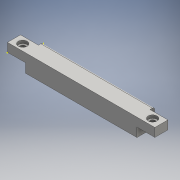
# Autodesk Inventor part: beam44mmVer2
Saved by Autodesk Inventor 2016 (Build 200138000, 138)
## iProperties
Created: 2015-11-25
Part Number: beam44mmVer2
Material: Generic
Document SubType Name: Modeling
Designer: hesaon
Density: 1 g/cm^3
Appearance: Default
Author: hesaon
Autodesk Inventor part; units mm, degrees
ref_plane "YZ Plane" through (0, 0, 0) normal (1, 0, 0) x (0, 1, 0)
ref_plane "XZ Plane" through (0, 0, 0) normal (0, 1, 0) x (-1, 0, 0)
ref_plane "XY Plane" through (0, 0, 0) normal (0, 0, 1) x (1, 0, 0)
sketch "Sketch1" plane through (0, 0, 0) normal (0, 0, 1) x (1, 0, 0)
  line L0 (0, 0) -> (100, 0)
  line L1 (100, 0) -> (100, 8.85)
  line L2 (87.85, 12) -> (12.15, 12)
  line L3 (0, 8.85) -> (0, 0)
  line L4 (12.15, 12) -> (12.15, 8.85)
  line L5 (12.15, 8.85) -> (0, 8.85)
  line L6 (87.85, 12) -> (87.85, 8.85)
  line L7 (87.85, 8.85) -> (100, 8.85)
  dimension "d6" = 100
  dimension "d7" = 3.15
  dimension "d8" = 3.15
  dimension "d9" = 12.15
  dimension "d10" = 12.15
  dimension "d11" = 8.85
  dimension "d12" = 8.85
  dimension "d13" = 12
  constraints: 16 end point, 2 parallel, 1 horizontal, 1 perpendicular
  measures "d6" distance of L0.end L0.start
  measures "d7" distance of L2.end L4.end
  measures "d8" distance of L6.end L2.start
  measures "d9" distance between parallel lines of L4 L3
  measures "d10" distance between parallel lines of L1 L6
  measures "d11" distance of L3.start L0.start
  measures "d12" distance of L1.end L0.end
  measures "d13" distance from line of L0 L2.end
extrude "Extrusion1" add sketch "Sketch1" along normal blind 6
sketch "Sketch2" plane through (0, 0, 0) normal (0, 0, -1) x (-1, 0, 0)
  line L0 (-87.85, 12) -> (-12.15, 12) projected
  line L1 (0, 0) -> (-100, 0) projected
  line L2 (-87.85, 12) -> (-12, 12)
  line L3 (-12, 12) -> (-12, 0)
  line L4 (-12, 0) -> (-87.85, 0)
  line L5 (-87.85, 0) -> (-87.85, 12)
  constraints: 8 end point, 2 parallel, 1 horizontal, 1 perpendicular, 1 point on line
extrude "Extrusion2" add sketch "Sketch2" along normal blind 6
sketch "Sketch3" plane through (0, 0, 0) normal (0, 0, -1) x (-1, 0, 0)
  circle A0 centre (-6, 4.35) radius 1.725
  line L0 (-12, 8.85) -> (0, 8.85) projected
  line L1 (0, 8.85) -> (0, 0) projected
  circle A1 centre (-94, 4.5) radius 1.725
  line L2 (-87.85, 0) -> (-100, 0) projected
  line L3 (-100, 0) -> (-100, 8.85) projected
  point P0 (-12, 9)
  dimension "d18" = 3.45
  dimension "d19" = 4.5
  dimension "d20" = 6
  dimension "d21" = 3.45
  dimension "d22" = 4.5
  dimension "d23" = 6
  constraints: 2 centre point, 1 other
  measures "d18" diameter of A0
  measures "d20" distance from line of L1 A0.centre
  measures "d21" diameter of A1
  measures "d22" distance from line of L2 A1.centre
  measures "d23" distance from line of L3 A1.centre
extrude "Extrusion3" cut sketch "Sketch3" against normal blind 4
sketch "Sketch4" plane through (0, 0, 6) normal (0, 0, 1) x (1, 0, 0)
  circle A0 centre (6, 4.35) radius 3
  line L0 (12.15, 8.85) -> (0, 8.85) projected
  line L1 (0, 8.85) -> (0, 0) projected
  circle A1 centre (94, 4.5) radius 1.725 projected
  circle A2 centre (94, 4.5) radius 3
  dimension "d26" = 6
  dimension "d27" = 4.5
  dimension "d28" = 6
  dimension "d29" = 6
  constraints: 2 centre point, 1 coincident
  measures "d26" diameter of A0
  measures "d27" distance from line of L0 A0.centre
  measures "d28" distance from line of L1 A0.centre
  measures "d29" diameter of A2
extrude "Extrusion4" cut sketch "Sketch4" against normal blind 2 contours A0 | A1 | A2
sketch "Sketch5" plane through (87.85, 0, 0) normal (0, -1, 0) x (1, 0, 0)
  point P0 (-87.85, 0)
sketch "Sketch6" plane through (0, 0, 0) normal (0, 0, -1) x (-1, 0, 0)
  line L0 (0, 0) -> (-100, 0) projected
  line L1 (-12.15, 8.85) -> (0, 8.85) projected
  line L2 (0, 0) -> (0, 8.85)
  line L3 (-12.15, 8.85) -> (-12, 8.85) projected
  line L4 (0, 8.85) -> (-12, 8.85)
  line L5 (-12, 0) -> (-12, 12) projected
  line L6 (-12, 8.85) -> (-12, 0)
  line L7 (-12, 0) -> (0, 0)
  line L8 (-100, 0) -> (-100, 8.85) projected
  line L9 (-100, 0) -> (-87.85, 0)
  line L10 (-87.85, 0) -> (-87.85, 8.85) projected
  line L11 (-87.85, 0) -> (-87.85, 8.85)
  line L12 (-87.85, 8.85) -> (-100, 8.85)
  line L13 (-100, 8.85) -> (-100, 0)
  dimension "d33" = 12.15
  constraints: 16 end point, 5 collinear, 1 perpendicular, 1 point on line, 1 vertical
  measures "d33" distance of L0.end L9.end
extrude "Extrusion5" cut sketch "Sketch6" against normal blind 0.15
sketch "Sketch7" plane through (12, 8.85, 0) normal (-1, 0, 0) x (0, 0, 1)
  line L0 (0, 3.15) -> (0, 0) projected
  line L1 (0, 3.15) -> (0, 0)
  line L2 (0.15, 0) -> (6, 0) projected
  line L3 (0, 0) -> (0.15, 0)
  line L4 (0.15, 0) -> (0.15, -8.85) projected
  line L5 (0.15, 0) -> (0.15, -8.85)
  line L6 (0.15, -8.85) -> (-6, -8.85) projected
  line L7 (0.15, -8.85) -> (-6, -8.85)
  line L8 (-6, -8.85) -> (-6, 3.15)
  line L9 (0, 3.15) -> (6, 3.15) projected
  line L10 (-6, 3.15) -> (0, 3.15)
  point P0 (0, -8.85)
  constraints: 12 end point, 3 collinear, 3 perpendicular
sketch "Sketch8" plane through (12.15, 12, 6) normal (0, 1, 0) x (1, 0, 0)
  line L0 (0, 6) -> (0, 0) projected
  line L1 (75.7, 12) -> (-0.15, 12) projected
  line L2 (0, 6) -> (-0.15, 6)
  line L3 (-0.15, 6) -> (-0.15, 12)
  line L4 (-0.15, 12) -> (0, 12)
  line L5 (0, 12) -> (0, 6)
  point P0 (-12.15, 6)
  constraints: 8 end point, 2 parallel, 1 horizontal, 1 perpendicular
extrude "Extrusion6" cut sketch "Sketch7" against normal blind 0.15
fillet "Fillet2" radius 1.5 2 edges at (50, 12, 6) (50, 12, -6)
equation "\"d8\" = d7"
equation "\"d10\" = d9"
equation "\"d12\" = d11"
body "Solid1"
